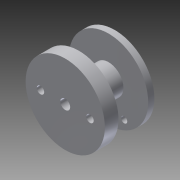
# Autodesk Inventor part: Girouette
Saved by Autodesk Inventor 2014 SP2 (Build 180246200, 246)
## iProperties
Created: 2014-10-15
Part Number: Girouette
Material: Plastique ABS
Document SubType Name: Modeling
Designer: sd
Density: 1.06 g/cm^3
Appearance: Lisse - Blanc
Author: sd
Autodesk Inventor part; units mm, degrees
ref_plane "YZ Plane" through (0, 0, 0) normal (1, 0, 0) x (0, 1, 0)
ref_plane "XZ Plane" through (0, 0, 0) normal (0, 1, 0) x (-1, 0, 0)
ref_plane "XY Plane" through (0, 0, 0) normal (0, 0, 1) x (1, 0, 0)
sketch "Esquisse1" plane through (0, 0, 0) normal (0, 1, 0) x (-1, 0, 0)
  circle A0 centre (0, 0) radius 16
  dimension "D" = 32
  constraints: 1 centre point, 1 coincident
  measures "D" diameter of A0
extrude "Extrusion1" add sketch "Esquisse1" along normal blind 5.5
sketch "Esquisse2" plane through (0, 5.5, 0) normal (0, 1, 0) x (1, 0, 0)
  circle A0 centre (0, 0) radius 16 projected
  circle A1 centre (0, 0) radius 6
  dimension "d3" = 12
  constraints: 1 centre point, 1 coincident
  measures "d3" diameter of A1
extrude "Extrusion2" add sketch "Esquisse2" along normal blind 12 contours A1
sketch "Esquisse4" plane through (0, 17.5, 0) normal (0, 1, 0) x (1, 0, 0)
  circle A0 centre (0, 0) radius 6 projected
  circle A1 centre (0, 0) radius 16
  dimension "d8" = 32
  constraints: 1 centre point, 1 coincident
  measures "d8" diameter of A1
extrude "Extrusion4" add sketch "Esquisse4" along normal blind 2.5 contours A0 | A1
sketch "Esquisse5" plane through (0, 20, 0) normal (0, 1, 0) x (1, 0, 0)
  circle A0 centre (0, 0) radius 16 projected
  circle A1 centre (0, 0) radius 2
  dimension "P" = 4
  constraints: 1 centre point, 1 coincident
  measures "P" diameter of A1
extrude "Extrusion5" cut sketch "Esquisse5" against normal through all contours A1
sketch "Esquisse6" plane through (0, 0, 0) normal (0, -1, 0) x (1, 0, 0)
  circle A0 centre (0, 0) radius 2 projected
  circle A1 centre (-10, 0) radius 1.5
  circle A2 centre (10, 0) radius 1.5
  dimension "p2" = 3
  dimension "d15" = 3
  dimension "d16" = 20
  dimension "d17" = 10
  constraints: 2 centre point
  measures "p2" diameter of A1
  measures "d15" diameter of A2
  measures "d16" distance of A2.centre A1.centre
  measures "d17" distance of A0.centre A1.centre
extrude "Extrusion6" cut sketch "Esquisse6" against normal blind 5.5 contours A1 | A2
sketch "Esquisse7" plane through (0, 20, 0) normal (0, 1, 0) x (1, 0, 0)
  circle A0 centre (0, 0) radius 2 projected
  circle A1 centre (-6.3, 11) radius 1.25
  circle A2 centre (6.3, 11) radius 1.25
  dimension "e" = 2.5
  dimension "d21" = 12.6
  dimension "d22" = 6.3
  dimension "d23" = 11
  dimension "d24" = 2.5
  dimension "d25" = 11
  constraints: 2 centre point
  measures "e" diameter of A1
  measures "d21" distance of A2.centre A1.centre
  measures "d22" horizontal distance of A0.centre A1.centre
  measures "d23" vertical distance of A0.centre A1.centre
  measures "d24" diameter of A2
  measures "d25" vertical distance of A0.centre A2.centre
extrude "Extrusion7" cut sketch "Esquisse7" against normal blind 2.5 contours A1 | A2
equation "\"d8\" = D"
equation "\"d15\" = p2"
equation "\"d17\" = 0.5 * d16"
equation "\"d18\" = d1"
equation "\"d22\" = 0.5 * d21"
equation "\"d24\" = e"
equation "\"d25\" = d23"
equation "\"d1\" = 5.5"
